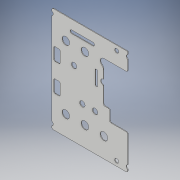
# Autodesk Inventor part: End Plate - 18S
Saved by Autodesk Inventor 2017 (Build 210142000, 142)
## iProperties
Created: 2021-03-03
Part Number: End Plate - 18S
Material: Generic
Document SubType Name: Modeling
Designer: Win240
Density: 1 g/cm^3
Appearance: Default
Author: Win240
Autodesk Inventor part; units mm, degrees
ref_plane "YZ Plane" through (0, 0, 0) normal (1, 0, 0) x (0, 1, 0)
ref_plane "XZ Plane" through (0, 0, 0) normal (0, 1, 0) x (-1, 0, 0)
ref_plane "XY Plane" through (0, 0, 0) normal (0, 0, 1) x (1, 0, 0)
sketch "Sketch1" plane through (0, 0, 0) normal (0, 0, 1) x (1, 0, 0)
  line L0 (0, 0) -> (119, 0)
  line L1 (119, 0) -> (119, -28)
  line L2 (119, -165) -> (0, -165)
  line L3 (0, -165) -> (0, 0)
  arc A0 (0, -10.5923) -> (0, -4.4077) centre (-1, -7.5) ccw
  arc A1 (119, -4.4077) -> (119, -10.5923) centre (120, -7.5) ccw
  arc A2 (119, -154.4077) -> (119, -160.5923) centre (120, -157.5) ccw
  arc A3 (0, -160.5923) -> (0, -154.4077) centre (-1, -157.5) ccw
  line L4 (-1, -7.5) -> (120, -7.5) construction
  line L5 (120, -7.5) -> (120, -157.5) construction
  line L6 (120, -157.5) -> (-1, -157.5) construction
  line L7 (-1, -157.5) -> (-1, -7.5) construction
  line L8 (-1, -7.5) -> (0, -4.4077) construction
  line L9 (120, -7.5) -> (119, -4.4077) construction
  line L10 (59.5, -7.5) -> (59.5, 0) construction
  line L11 (59.5, -157.5) -> (59.5, -165) construction
  circle A4 centre (22, -34) radius 6
  circle A5 centre (52, -34) radius 6
  arc A6 (82, -28) -> (78.5, -38.8734) centre (82, -34) ccw
  circle A7 centre (82, -134) radius 6
  circle A8 centre (52, -134) radius 6
  circle A9 centre (22, -134) radius 6
  line L12 (22, -34) -> (52, -34) construction
  line L13 (52, -34) -> (82, -34) construction
  line L14 (82, -34) -> (82, -134) construction
  line L15 (82, -134) -> (52, -134) construction
  line L16 (52, -134) -> (22, -134) construction
  line L17 (22, -134) -> (22, -34) construction
  circle A10 centre (68, -107) radius 4.25
  circle A11 centre (35, -61) radius 4.25
  circle A12 centre (102, -7.5) radius 3.25
  line L18 (68, -48.5) -> (72, -48.5)
  line L19 (72, -48.5) -> (72, -72.5)
  line L20 (72, -72.5) -> (68, -72.5)
  line L21 (68, -72.5) -> (68, -48.5)
  line L22 (82, -28) -> (119, -28)
  line L23 (81, -43.7468) -> (81, -92.5)
  arc A13 (81, -56.75) -> (81, -65.25) centre (81, -61) ccw
  circle A14 centre (48, -107) radius 4.25
  line L24 (48, -107) -> (68, -107) construction
  line L25 (35, -61) -> (81, -61) construction
  arc A15 (81, -43.7468) -> (78.5, -38.8734) centre (75, -43.7468) ccw
  line L26 (81, -92.5) -> (91, -92.5)
  line L27 (91, -92.5) -> (91, -110.5)
  line L28 (91, -110.5) -> (119, -110.5)
  arc A16 (82, -40) -> (82, -28) centre (82, -34) ccw construction
  arc A17 (78.5, -38.8734) -> (82, -40) centre (82, -34) ccw construction
  arc A18 (82, -56.8693) -> (81, -56.75) centre (81, -61) ccw construction
  arc A19 (82, -65.1307) -> (82, -56.8693) centre (81, -61) ccw construction
  arc A20 (81, -65.25) -> (82, -65.1307) centre (81, -61) ccw construction
  line L29 (119, -28) -> (119, -110.5) construction
  line L30 (119, -110.5) -> (119, -165)
  circle A21 centre (102, -157.5) radius 3.25
  line L31 (102, -7.5) -> (102, -157.5) construction
  dimension "d0" = 119
  dimension "d1" = 165
  dimension "d2" = 150
  dimension "d3" = 121
  dimension "d4" = 3.25
  dimension "d5" = 12
  dimension "d6" = 30
  dimension "d7" = 100
  dimension "d8" = 26.5
  dimension "d9" = 23
  dimension "d10" = 8.5
  dimension "d11" = 36
  dimension "d12" = 69
  dimension "d13" = 53.5
  dimension "d14" = 99.5
  dimension "d15" = 103
  dimension "d16" = 65
  dimension "d17" = 41
  dimension "d18" = 69
  dimension "d19" = 73
  dimension "d20" = 82
  dimension "d21" = 82
  dimension "d22" = 49
  dimension "d23" = 85
  dimension "d24" = 92
  dimension "d25" = 103
  constraints: 64 end point, 24 point on circle, 22 centre point, 20 point on line, 14 equal radius, 13 horizontal, 8 vertical, 6 parallel, 4 midpoint, 4 perpendicular, 4 tangent, 3 equal length
  measures "d0" distance of L2.start L2.end
  measures "d1" distance of L0.end L2.start
  measures "d2" distance of L4.end L5.end
  measures "d3" distance of L5.end L6.end
  measures "d4" radius of A0
  measures "d5" diameter of A4
  measures "d6" distance of L12.start L12.end
  measures "d7" distance of L16.end L12.start
  measures "d8" distance between parallel lines of L4 L12
  measures "d9" distance between parallel lines of L17 L7
  measures "d10" diameter of A11
  measures "d11" distance from line of L25.start L7
  measures "d12" distance from line of L24.end L7
  measures "d13" distance from line of L25.start L4
  measures "d14" distance from line of L4 L24.end
  measures "d15" distance of L31.start L4.start
  measures "d16" distance between parallel lines of L20 L4
  measures "d17" distance between parallel lines of L18 L4
  measures "d18" distance between parallel lines of L21 L7
  measures "d19" distance between parallel lines of L19 L7
  measures "d20" distance between parallel lines of L7 L23
  measures "d21" distance from line of L7 L25.end
  measures "d22" distance from line of L24.start L7
  measures "d23" distance between parallel lines of L4 L26
  measures "d24" distance between parallel lines of L7 L27
  measures "d25" distance between parallel lines of L4 L28
extrude "Mechanical Holes" add sketch "Sketch1" along normal blind 1 contours L0 L1 A1 L22 A6 A15 L23 A13 L26 L27 L28 L30 A2 L2 L3 A3 A0
sketch "Sketch2" plane through (0, 0, 1) normal (0, 0, 1) x (1, 0, 0)
  line L0 (0, -10.5923) -> (0, -154.4077) projected
  line L1 (119, 0) -> (0, 0) projected
  line L2 (0, -165) -> (119, -165) projected
  line L3 (67, -14.5) -> (29, -14.5)
  line L4 (29, -14.5) -> (29, -19.5)
  line L5 (29, -19.5) -> (67, -19.5)
  line L6 (67, -19.5) -> (67, -14.5)
  line L7 (3, -50.5) -> (13, -50.5)
  line L8 (13, -50.5) -> (13, -70.5)
  line L9 (13, -70.5) -> (3, -70.5)
  line L10 (3, -70.5) -> (3, -50.5)
  arc A0 (0, -10.5923) -> (0, -4.4077) centre (-1, -7.5) ccw construction
  line L11 (13, -94.5) -> (3, -94.5)
  line L12 (3, -94.5) -> (3, -114.5)
  line L13 (3, -114.5) -> (13, -114.5)
  line L14 (13, -114.5) -> (13, -94.5)
  dimension "d28" = 4
  dimension "d29" = 10
  dimension "d30" = 63
  dimension "d31" = 87
  dimension "d32" = 20
  dimension "d33" = 7
  dimension "d34" = 12
  dimension "d35" = 30
  dimension "d36" = 68
  constraints: 24 end point, 6 parallel, 3 collinear, 3 horizontal, 3 perpendicular
  measures "d28" distance from line of L10 A0.centre
  measures "d29" distance of L7.start L7.end
  measures "d30" distance from line of L9 A0.centre
  measures "d31" distance from line of L11 A0.centre
  measures "d32" distance of L7.end L8.end
  measures "d33" distance from line of A0.centre L3
  measures "d34" distance from line of A0.centre L5
  measures "d35" distance from line of L4 A0.centre
  measures "d36" distance from line of A0.centre L6
extrude "Air Holes" cut sketch "Sketch2" against normal up to surface (1 mm away)
fillet "Fillet1" radius 2 24 edges at (119, -28, 0.5) (81, -92.5, 0.5) (91, -92.5, 0.5) (91, -110.5, 0.5) (119, -110.5, 0.5) (119, -165, 0.5) (0, -165, 0.5) (13, -94.5, 0.5) (13, -114.5, 0.5) (3, -114.5, 0.5) (3, -94.5, 0.5) (3, -50.5, 0.5) (29, -14.5, 0.5) (68, -48.5, 0.5) (72, -48.5, 0.5) (67, -14.5, 0.5) (13, -50.5, 0.5) (72, -72.5, 0.5) (13, -70.5, 0.5) (67, -19.5, 0.5) (68, -72.5, 0.5) (29, -19.5, 0.5) (3, -70.5, 0.5) (0, 0, 0.5)
body "Solid1"
